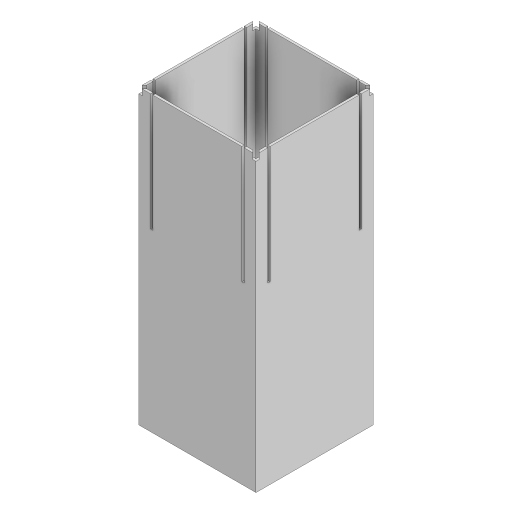
# Autodesk Inventor part: FLueExtension
Saved by Autodesk Inventor 2024.3 (Build 283343000, 343)
## iProperties
Created: 2025-09-16
Part Number: FLueExtension
Material: Generic
Document SubType Name: Modeling
Designer: ajclo
Density: 1 g/cm^3
Appearance: Default
Author: ajclo
Autodesk Inventor part; units mm, degrees
ref_plane "YZ Plane" through (0, 0, 0) normal (1, 0, 0) x (0, 1, 0)
sketch "Sketch1" plane through (0, 0, 0) normal (0, 1, 0) x (-1, 0, 0)
  line L0 (-50, 50) -> (50, 50)
  line L1 (50, 50) -> (50, -50)
  line L2 (50, -50) -> (-50, -50)
  line L3 (-50, -50) -> (-50, 50)
  line L4 (-50, 50) -> (50, -50) construction
  line L5 (50, 50) -> (-50, -50) construction
  line L6 (-48, 48) -> (48, 48)
  line L7 (48, 48) -> (48, -48)
  line L8 (48, -48) -> (-48, -48)
  line L9 (-48, -48) -> (-48, 48)
  line L10 (-48, 48) -> (48, -48) construction
  line L11 (48, 48) -> (-48, -48) construction
  point P0 (0, 0)
  dimension "d0" = 100
  dimension "d1" = 100
  dimension "d2" = 2
  constraints: 24 end point, 4 midpoint, 4 parallel, 2 horizontal, 2 perpendicular, 1 point on line
  measures "d0" distance of L0.end L1.end
  measures "d1" distance of L1.end L2.end
  measures "d2" distance between parallel lines of L2 L8
extrude "Extrusion1" add sketch "Sketch1" along normal blind 250
sketch "Sketch3" plane through (50, 250, 50) normal (1, 0, 0) x (0, 0, -1)
  line L0 (2, 0) -> (98, 0) projected
  line L1 (10, 0) -> (12, 0)
  line L2 (12, 0) -> (12, -100)
  line L3 (12, -100) -> (10, -100)
  line L4 (10, -100) -> (10, 0)
  line L5 (0, -250) -> (0, 0) projected
  point P0 (50, -250)
  point P1 (0, -146)
  point P2 (12, 0)
  dimension "d9" = 100
  dimension "d10" = 2
  dimension "d11" = 10
  constraints: 8 end point, 2 parallel, 1 horizontal, 1 perpendicular, 1 point on line
  measures "d9" distance of L1.end L2.end
  measures "d10" distance between parallel lines of L2 L4
  measures "d11" distance between parallel lines of L5 L4
extrude "Extrusion3" cut sketch "Sketch3" against normal blind 220
mirror "Mirror2" about plane through (0, 0, 0) normal (0, 0, 1) of "Extrusion3"
sketch "Sketch4" plane through (-50, 250, 50) normal (0, 0, 1) x (1, 0, 0)
  line L0 (10, 0) -> (12, 0)
  line L1 (12, 0) -> (12, -100)
  line L2 (12, -100) -> (10, -100)
  line L3 (10, -100) -> (10, 0)
  line L4 (0, -250) -> (0, 0) projected
  line L5 (0, 0) -> (100, 0) projected
  point P0 (50, -250)
  point P1 (0, -146)
  point P2 (10, -50)
  point P3 (11, 0)
  dimension "d14" = 10
  dimension "d15" = 2
  dimension "d16" = 100
  dimension "d17" = 0
  constraints: 8 end point, 2 midpoint, 2 parallel, 1 horizontal, 1 perpendicular
  measures "d14" distance between parallel lines of L4 L3
  measures "d15" distance from line of L1 point (10, -50)
  measures "d16" distance of L0.end L1.end
  measures "d17" distance from line of L5 point (11, 0)
extrude "Extrusion4" cut sketch "Sketch4" against normal blind 220
mirror "Mirror3" about plane through (0, 0, 0) normal (1, 0, 0) of "Extrusion4"
ref_plane "Work Plane1" through (50, 104, 50) normal (-0.7071, 0, 0.7071) x (0, -1, 0)
sketch "Sketch5" plane through (50, 104, 50) normal (-0.7071, 0, 0.7071) x (0, -1, 0)
  line L0 (-141, -72.7107) -> (-146, -72.7107)
  line L1 (-146, -72.7107) -> (-146, -68.7107)
  line L2 (-146, -68.7107) -> (-141, -68.7107)
  line L3 (-141, -68.7107) -> (-141, -72.7107)
  line L4 (-141, -72.7107) -> (-146, -68.7107) construction
  line L5 (-146, -72.7107) -> (-141, -68.7107) construction
  line L6 (104, -70.7107) -> (-146, -70.7107) projected
  point P0 (-143.5, -70.7107)
  point P1 (0, -70.7107)
  dimension "d20" = 5
  dimension "d21" = 4
  dimension "d22" = 0
  dimension "d23" = 0
  constraints: 12 end point, 3 midpoint, 2 parallel, 1 horizontal, 1 perpendicular
  measures "d20" distance of L1.end L2.end
  measures "d21" distance between parallel lines of L2 L0
  measures "d22" distance from line of L6 point (-143.5, -70.711)
  measures "d23" distance of L6.end point (-146, -70.711)
extrude "Extrusion5" cut sketch "Sketch5" along normal mid plane 220
ref_plane "Work Plane2" through (-48, 104, 50) normal (0.7071, 0, 0.7071) x (0, 1, 0)
sketch "Sketch6" plane through (-48, 104, 50) normal (0.7071, 0, 0.7071) x (0, 1, 0)
  line L0 (141, -67.2965) -> (146, -67.2965)
  line L1 (146, -67.2965) -> (146, -71.2965)
  line L2 (146, -71.2965) -> (141, -71.2965)
  line L3 (141, -71.2965) -> (141, -67.2965)
  line L4 (-104, -69.2965) -> (146, -69.2965) projected
  line L5 (141, -67.2965) -> (146, -71.2965) construction
  line L6 (146, -67.2965) -> (141, -71.2965) construction
  line L7 (146, -62.2254) -> (146, -69.2965) projected
  point P0 (143.5, -69.2965)
  point P1 (0, -69.2965)
  dimension "d26" = 4
  dimension "d27" = 5
  dimension "d28" = 0
  constraints: 12 end point, 2 midpoint, 2 parallel, 1 horizontal, 1 perpendicular, 1 point on line
  measures "d26" distance between parallel lines of L2 L0
  measures "d27" distance of L1.end L2.end
  measures "d28" distance between parallel lines of L7 L1
extrude "Extrusion6" cut sketch "Sketch6" along normal mid plane 220
body "Solid1"
